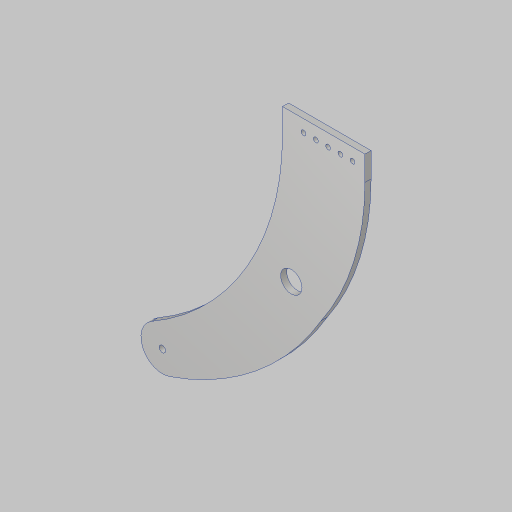
# Autodesk Inventor part: CL7-008
Saved by Autodesk Inventor 2023.5 (Build 275446000, 446)
## iProperties
Created: 2025-03-17
Part Number: CL7-008
Material: Aluminum 6061
Document SubType Name: Modeling
Designer: slick
Density: 2.7 g/cm^3
Appearance: Aluminum - Flat
Author: slick
Autodesk Inventor part; units mm, degrees
ref_plane "YZ Plane" through (0, 0, 0) normal (1, 0, 0) x (0, 1, 0)
ref_plane "XZ Plane" through (0, 0, 0) normal (0, 1, 0) x (-1, 0, 0)
ref_plane "XY Plane" through (0, 0, 0) normal (0, 0, 1) x (1, 0, 0)
sketch "Sketch1" plane through (0, 0, 0) normal (0, 0, 1) x (1, 0, 0)
  line L0 (-146.05, 152.4) -> (76.2, 152.4) construction
  line L1 (76.2, 152.4) -> (76.2, 127) construction
  line L2 (76.2, 127) -> (-146.05, 127) construction
  line L3 (-146.05, 127) -> (-146.05, 152.4) construction
  circle A0 centre (-133.35, -127) radius 12.7 construction
  circle A1 centre (0, 0) radius 23.8125 construction
  circle A2 centre (0, 0) radius 11.1125
  circle A3 centre (0, 0) radius 36.5125 construction
  line L4 (76.2, 152.4) -> (76.2, 127)
  line L5 (76.2, 152.4) -> (-9.0845, 152.4)
  line L6 (-9.0845, 152.4) -> (-9.0845, 127)
  circle A4 centre (-133.35, -127) radius 22.225 construction
  arc A5 (-144.4803, -107.7629) -> (-9.0845, 127) centre (-280.3101, 127) ccw
  arc A6 (-126.1231, -148.0172) -> (31.5864, -18.3156) centre (-221.1051, 128.2089) ccw
  arc A7 (-144.4803, -107.7629) -> (-126.1231, -148.0172) centre (-133.35, -127) ccw
  arc A8 (30.0156, -20.79) -> (76.2, 127) centre (-183.3562, 127) ccw
  arc A9 (31.5864, -18.3156) -> (30.9373, -19.3918) centre (0, 0) ccw
  line L7 (-69.85, 152.4) -> (-69.85, 127) construction
  point P0 (63.5, 139.7)
  point P1 (76.2, 139.7)
  point P2 (50.8, 139.7)
  point P3 (38.1, 139.7)
  point P4 (25.4, 139.7)
  point P5 (12.7, 139.7)
  point P6 (30.0156, -20.79)
  point P7 (-33.2582, 15.0683)
  point P8 (30.851, -19.5766)
  point P9 (-69.85, 139.7)
  dimension "d0" = 25.4
  dimension "d1" = 127
  dimension "d2" = 222.25
  dimension "d3" = 146.05
  dimension "d4" = 25.4
  dimension "d5" = 127
  dimension "d7" = 12.7
  dimension "d8" = 47.625
  dimension "d9" = 22.225
  dimension "d12" = 12.7
  dimension "d17" = 12.7
  dimension "d18" = 9.525
  dimension "d19" = 292.1
  dimension "d37" = 146.05
  dimension "d38" = 63.5
  constraints: 16 end point, 15 point on circle, 10 centre point, 7 tangent, 5 coincident, 4 point on line, 3 perpendicular, 2 horizontal, 2 midpoint, 2 parallel, 1 horizontal alignment, 1 vertical, 4 other
  measures "d0" distance of L2.end L0.start
  measures "d1" distance from line of point (0, 0) L2
  measures "d2" distance of L0.start L0.end
  measures "d3" distance from line of point (0, 0) L3
  measures "d4" diameter of A0
  measures "d5" vertical distance of A0.centre point (0, 0)
  measures "d7" distance from line of L1 point (63.5, 139.7)
  measures "d8" diameter of A1
  measures "d9" diameter of A2
  measures "d12" distance of point (63.5, 139.7) point (50.8, 139.7)
  measures "d17" radial gap between concentric circles of A1 A3
  measures "d18" radial gap between concentric circles of A0 A4
  measures "d19" radius of A6
  measures "d37" distance from line of L0.end L7
  measures "d38" horizontal distance of point (-133.35, -127) point (-69.85, 139.7)
extrude "Extrusion1" add sketch "Sketch1" along normal blind 6.35
hole "Hole1" at (63.5, 139.7, 0) at (50.8, 139.7, 0) at (38.1, 139.7, 0) at (25.4, 139.7, 0) at (12.7, 139.7, 0) direction (0, 0, 1) diameter 5.1054 end through all clearance for "Flat Head Machine Screw (82)" size "#10" standard "Ansi Unified Screw Threads"
hole "Hole2" at (-133.35, -127, 0) direction (0, 0, 1) diameter 6.7564 end through all clearance for "Flat Head Machine Screw (82)" size "1/4" standard "Ansi Unified Screw Threads"
body "Solid1"
